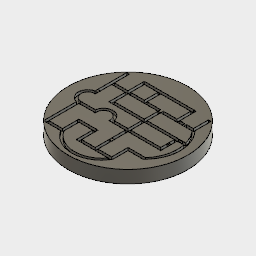
Maze_completed (Autodesk Fusion 360 design; units mm, degrees)
Autodesk Fusion 360 part; units mm, degrees
note: some values were not read from the file. Set by a fixed rule: which sketch regions a step uses.
(part 1 of 2)
sketch "Sketch1" plane through (0, 0, 0) normal (0, 1, 0) x (1, 0, 0)
  circle A0 centre (0, 0) radius 152.4
extrude "Extrude1" add sketch "Sketch1" along normal blind 25.4 makes body 1
sketch "Sketch2" plane through (0, 25.4, 0) normal (0, 1, 0) x (-1, 0, 0)
  circle A0 centre (0, 0) radius 152.4
  line L0 (62.5721, -104.2868) -> (62.572, -20.8574)
  line L1 (62.572, -20.8574) -> (-20.8574, -20.8574)
  line L2 (-20.8574, -20.8574) -> (-20.8574, 20.8573)
  line L3 (-20.8574, 20.8573) -> (20.8573, 20.8573)
  line L4 (62.572, 20.8573) -> (104.2868, 20.8573)
  line L5 (104.2868, 20.8573) -> (104.2868, 62.572)
  line L6 (104.2868, 62.572) -> (104.2868, 104.287)
  line L7 (104.2868, 104.287) -> (62.5718, 104.2869)
  line L8 (-62.5723, 104.2867) -> (-62.5722, 62.572)
  line L9 (-62.5722, 62.572) -> (-104.2867, 62.572)
  arc A1 (-104.2867, 62.572) -> (-104.2867, -62.5721) centre (-41.0104, -0.0001) ccw
  arc A2 (20.8573, 20.8573) -> (62.572, 20.8573) centre (41.7146, 20.7869) ccw
  line L10 (104.2868, -104.2868) -> (104.2868, -20.8574)
  line L11 (20.8572, 62.572) -> (20.8571, 104.2868)
  line L12 (62.5719, 62.572) -> (20.8572, 62.572)
  line L13 (62.5718, 104.2869) -> (62.5719, 62.572)
  line L14 (20.8571, 104.2868) -> (-62.5723, 104.2867)
  line L15 (62.5721, -62.5721) -> (20.8574, -62.5721)
  line L16 (20.8574, -62.5721) -> (20.8574, -104.2868)
  line L17 (20.8574, -104.2868) -> (-20.8573, -104.2868)
  line L18 (-20.8573, -104.2868) -> (-62.572, -104.2868)
  line L19 (-104.2867, -62.5721) -> (-104.2867, -104.2868)
  line L20 (-104.2867, -62.5721) -> (-62.5721, -62.5721)
  line L21 (-62.5721, -62.5721) -> (-20.8573, -62.5721)
  line L22 (-20.8573, -62.5721) -> (-20.8574, -20.8574)
  line L23 (-20.8574, -20.8574) -> (-104.2867, -20.8574)
  line L24 (-104.2867, -20.8574) -> (-127.5212, -20.8575)
  line L25 (-20.8575, 62.572) -> (-20.8574, 20.8573)
  line L26 (-20.8575, 62.572) -> (-20.8576, 104.2868)
  line L27 (-62.5721, 20.8573) -> (-20.8574, 20.8573)
  line L28 (-104.2867, 20.8573) -> (-62.5721, 20.8573)
  line L29 (-104.2867, -20.8574) -> (-104.2867, 20.8573)
  arc A3 (104.2868, -20.8574) -> (104.2868, 20.8573) centre (102.4601, -0.0001) ccw
  line L30 (104.2868, -62.5721) -> (62.5721, -62.5721)
  arc A4 (62.5718, 104.2869) -> (-62.5723, 104.2867) centre (-0.0002, 67.3281) ccw
  circle A5 centre (123.3973, -0.0001) radius 7.4836
  circle A6 centre (-0.0003, 140) radius 10
  circle A7 centre (-104.2867, -0.0001) radius 7.4484
  line L31 (62.5721, -104.2868) -> (20.8574, -104.2868)
  line L32 (-62.572, -104.2868) -> (-62.5721, -62.5721)
  circle A8 centre (-20.8575, 83.4294) radius 6.8677
  circle A9 centre (-83.4294, -62.5721) radius 5.1809
  circle A10 centre (-115.9039, -20.8575) radius 5.6269
  line L33 (20.8574, -62.5721) -> (-20.8573, -62.5721)
  circle A11 centre (-20.8573, -62.5721) radius 8.2188
  line L34 (104.2868, -104.2868) -> (100.9118, -104.2868)
  line L35 (104.2868, -104.2868) -> (107.6618, -104.2868)
  line L36 (100.9118, -104.2868) -> (100.9118, -62.5721)
  line L37 (107.6618, -104.2868) -> (107.6618, -20.2808)
  line L38 (104.2868, -62.5721) -> (104.2868, -65.9471)
  line L39 (104.2868, -62.5721) -> (104.2868, -59.1971)
  line L40 (104.2868, -65.9471) -> (62.5721, -65.9472)
  line L41 (104.2868, -59.1971) -> (62.5721, -59.1972)
  line L42 (100.9118, -62.5721) -> (100.9118, -20.7212)
  line L43 (62.5721, -62.5721) -> (65.9471, -62.5721)
  line L44 (62.5721, -62.5721) -> (59.1971, -62.5721)
  line L45 (59.1971, -62.5721) -> (59.1971, -104.2868)
  line L46 (65.9471, -62.5721) -> (65.9472, -104.2868)
  line L47 (65.9472, -104.2868) -> (62.5721, -104.2868)
  line L48 (59.1971, -62.5721) -> (59.1971, -20.8574)
  line L49 (65.9471, -62.5721) -> (65.9472, -83.4295)
  line L50 (62.572, -20.8574) -> (65.947, -20.8574)
  line L51 (65.9471, -62.5721) -> (65.947, -20.8574)
  line L52 (104.2868, -20.8574) -> (100.9118, -20.8574)
  line L53 (104.2868, -20.8574) -> (104.2868, -24.2324)
  line L54 (104.2868, -20.8574) -> (104.2868, -17.4824)
  line L55 (104.2868, 20.8573) -> (104.2868, 17.4823)
  line L56 (104.2868, 20.8573) -> (104.2868, 24.2323)
  line L57 (123.3973, -0.0001) -> (126.7723, -0.0001)
  arc A12 (104.2868, -24.2324) -> (104.2868, 24.2323) centre (102.4721, -0.0001) ccw
  line L58 (123.3973, -0.0001) -> (120.0223, -0.0001)
  arc A13 (104.2868, -17.4824) -> (104.2868, 17.4823) centre (102.443, -0.0001) ccw
  line L59 (65.9472, -104.2868) -> (65.9472, -100.9118)
  line L60 (65.9472, -104.2868) -> (65.9471, -107.6618)
  line L61 (-62.572, -104.2868) -> (-62.572, -107.6618)
  line L62 (-62.572, -104.2868) -> (-62.572, -100.9118)
  line L63 (65.9471, -107.6618) -> (-62.572, -107.6618)
  line L64 (-62.572, -100.9118) -> (65.9472, -100.9118)
  line L65 (20.8574, -104.2868) -> (24.2324, -104.2868)
  line L66 (20.8574, -104.2868) -> (17.4824, -104.2868)
  line L67 (17.4824, -104.2868) -> (17.4824, -62.5721)
  line L68 (24.2324, -104.2868) -> (24.2324, -62.5721)
  line L69 (62.5721, -65.9472) -> (20.8574, -65.9473)
  line L70 (20.8574, -62.5721) -> (20.8574, -59.1972)
  line L71 (20.8574, -59.1972) -> (62.5721, -59.1972)
  line L72 (20.8574, -59.1972) -> (-20.8573, -59.1973)
  line L73 (-20.8573, -62.5721) -> (-20.8574, -65.9474)
  line L74 (-20.8574, -65.9474) -> (20.8574, -65.9473)
  line L75 (-20.8574, -65.9474) -> (-104.2867, -65.9474)
  line L76 (-20.8573, -59.1973) -> (-104.2867, -59.1973)
  line L77 (-104.2867, -59.1973) -> (-104.2867, -62.5721)
  line L78 (-104.2867, -62.5721) -> (-107.6617, -62.5721)
  line L79 (-107.6617, -62.5721) -> (-107.6617, -104.2871)
  line L80 (-107.6617, -104.2871) -> (-104.2867, -104.2868)
  line L81 (-104.2867, -62.5721) -> (-100.9117, -62.5721)
  line L82 (-100.9117, -62.5721) -> (-100.9117, -104.287)
  line L83 (-100.9117, -104.287) -> (-104.2867, -104.2868)
  line L84 (-104.2867, -59.1973) -> (-107.6617, -59.1973)
  line L85 (-107.6617, -59.1973) -> (-107.6617, -62.5721)
  line L86 (-104.2867, 62.572) -> (-104.2867, 65.947)
  line L87 (-104.2867, -62.5721) -> (-104.2867, -66.5721)
  line L88 (-104.2867, -62.5721) -> (-104.2867, -58.5721)
  line L89 (-104.2867, 62.572) -> (-104.2867, 66.572)
  line L90 (-104.2867, 62.572) -> (-104.2867, 58.572)
  arc A14 (-100.9117, 62.572) -> (-100.9117, -62.5721) centre (-37.6354, -0.0001) ccw
  arc A15 (-107.6617, 62.572) -> (-107.6617, -62.5721) centre (-44.3854, -0.0001) ccw
  line L91 (65.947, -20.8574) -> (65.947, -24.2324)
  line L92 (65.947, -20.8574) -> (65.947, -17.4824)
  line L93 (65.947, -17.4824) -> (-104.2867, -17.4824)
  line L94 (65.947, -24.2324) -> (-104.2867, -24.2329)
  line L95 (-104.2867, -24.2329) -> (-104.2867, -20.8574)
  line L96 (-20.8574, -20.8574) -> (-17.4824, -20.8574)
  line L97 (-20.8574, -20.8574) -> (-24.2324, -20.8574)
  line L98 (-24.2324, -20.8574) -> (-24.2324, -62.5721)
  line L99 (-17.4824, -20.8574) -> (-17.4824, -62.5721)
  line L100 (-104.2867, -24.2329) -> (-123.262, -24.2329)
  line L101 (-104.2867, -17.4824) -> (-124.8909, -17.4824)
  line L102 (20.8573, 20.8573) -> (20.8573, 17.4823)
  line L103 (20.8573, 17.4823) -> (20.8573, 20.8573)
  line L104 (20.8573, 20.8573) -> (20.8573, 24.2323)
  line L105 (-104.2867, 20.8573) -> (-104.2867, 24.2323)
  line L106 (-104.2867, 24.2323) -> (20.8573, 24.2323)
  line L107 (20.8573, 17.4823) -> (-104.2867, 17.4823)
  line L108 (-104.2867, 24.2323) -> (-107.6617, 24.2323)
  line L109 (-107.6617, 24.2323) -> (-104.2867, 24.2323)
  line L110 (-104.2867, 24.2323) -> (-100.9117, 24.2323)
  line L111 (-100.9117, 24.2323) -> (-100.9117, -20.8574)
  line L112 (-107.6617, 24.2323) -> (-107.6616, -20.8574)
  line L113 (62.572, 20.8573) -> (62.572, 17.4823)
  line L114 (62.572, 17.4823) -> (62.572, 20.8573)
  line L115 (62.572, 20.8573) -> (62.5606, 24.2322)
  line L116 (62.5606, 24.2322) -> (104.2868, 24.2323)
  line L117 (104.2868, 17.4823) -> (62.572, 17.4823)
  line L118 (62.572, 20.8573) -> (65.947, 20.8573)
  line L119 (62.572, 20.8573) -> (59.197, 20.8573)
  line L120 (20.8573, 20.8573) -> (17.4823, 20.8573)
  line L121 (20.8573, 20.8573) -> (24.2323, 20.8573)
  line L122 (41.7146, -0.0706) -> (41.7146, 3.3044)
  line L123 (41.7146, 3.3044) -> (41.7146, -0.0706)
  line L124 (41.7146, -0.0706) -> (41.7146, -3.4456)
  arc A16 (17.4823, 20.8573) -> (65.947, 20.8573) centre (41.7146, 20.7869) ccw
  arc A17 (24.2323, 20.8573) -> (59.197, 20.8573) centre (41.7146, 20.7869) ccw
  line L125 (62.5606, 24.2322) -> (59.1856, 24.2322)
  line L126 (59.1856, 24.2322) -> (59.197, 20.8573)
  line L127 (24.2323, 20.8573) -> (24.2323, 24.2322)
  line L128 (24.2323, 24.2322) -> (20.8573, 24.2323)
  line L129 (-17.4824, -20.8574) -> (-17.4824, 20.8573)
  line L130 (-24.2324, -20.8574) -> (-24.2324, 20.8573)
  line L131 (-62.572, -107.6618) -> (-65.947, -107.6618)
  line L132 (-65.947, -107.6618) -> (-62.572, -107.6618)
  line L133 (-62.572, -107.6618) -> (-59.197, -107.6619)
  line L134 (-59.197, -107.6619) -> (-59.197, -65.9474)
  line L135 (-65.947, -107.6618) -> (-65.947, -65.9474)
  line L136 (104.2868, 104.287) -> (107.6618, 104.287)
  line L137 (107.6618, 104.287) -> (104.2868, 104.287)
  line L138 (104.2868, 104.287) -> (100.9118, 104.287)
  line L139 (107.6618, 104.287) -> (107.6618, 20.2806)
  line L140 (100.9118, 104.287) -> (100.9118, 24.2323)
  line L141 (107.6618, 104.287) -> (104.2868, 107.6568)
  line L142 (104.2868, 107.6568) -> (107.6618, 104.287)
  line L143 (62.5718, 104.2869) -> (62.5718, 100.9119)
  line L144 (62.5718, 100.9119) -> (104.2868, 100.9119)
  line L145 (104.2868, 107.6568) -> (60.4548, 107.6568)
  line L146 (62.5718, 104.2869) -> (59.1968, 104.2869)
  line L147 (59.1968, 104.2869) -> (62.5718, 104.2869)
  line L148 (62.5718, 104.2869) -> (65.9468, 104.2869)
  line L149 (-0.0003, 140) -> (-0.0003, 143.375)
  line L150 (-0.0003, 143.375) -> (-0.0003, 141.6875)
  line L151 (-0.0003, 140) -> (-0.0003, 136.625)
  line L152 (-62.5723, 104.2867) -> (-65.9473, 104.2867)
  line L153 (-62.5723, 104.2867) -> (-59.1973, 104.2867)
  arc A18 (65.9468, 104.2869) -> (-65.9473, 104.2867) centre (-0.0002, 68.2001) ccw
  arc A19 (59.1968, 104.2869) -> (-59.1973, 104.2867) centre (-0.0002, 66.274) ccw
  line L154 (62.5719, 62.572) -> (65.9469, 62.572)
  line L155 (65.9469, 62.572) -> (65.9468, 104.2869)
  line L156 (59.1968, 104.2869) -> (59.1969, 62.572)
  line L157 (65.9469, 62.572) -> (65.9469, 59.197)
  line L158 (65.9469, 59.197) -> (65.9469, 62.572)
  line L159 (65.9469, 62.572) -> (65.9469, 65.947)
  line L160 (20.8572, 62.572) -> (20.8571, 59.197)
  line L161 (65.9469, 59.197) -> (20.8571, 59.197)
  line L162 (65.9469, 65.947) -> (20.8572, 65.9469)
  line L163 (20.8571, 59.197) -> (17.4821, 59.197)
  line L164 (17.4821, 59.197) -> (17.4821, 104.2868)
  line L165 (20.8572, 62.572) -> (24.2322, 62.572)
  line L166 (24.2322, 62.572) -> (24.2322, 104.287)
  line L167 (24.2322, 104.287) -> (20.8571, 104.2868)
  line L168 (-17.4824, 20.8573) -> (-17.4825, 104.2868)
  line L169 (-24.2324, 20.8573) -> (-24.2324, 104.2868)
  line L170 (24.2322, 104.287) -> (24.2321, 107.662)
  line L171 (24.2322, 104.287) -> (24.2322, 100.912)
  line L172 (24.2322, 100.912) -> (-62.5723, 100.9118)
  line L173 (24.2321, 107.662) -> (-60.4537, 107.659)
  line L174 (-62.5722, 62.572) -> (-62.5722, 59.197)
  line L175 (-62.5722, 59.197) -> (-104.0798, 59.197)
  line L176 (-104.2867, 65.947) -> (-62.5722, 65.947)
  line L177 (-65.9473, 104.2867) -> (-65.9473, 59.197)
  line L178 (-62.5722, 59.197) -> (-59.1972, 59.197)
  line L179 (-59.1972, 59.197) -> (-59.1973, 104.2867)
  point P0 (62.5721, -104.2868)
  point P1 (62.5721, -62.5721)
  point P2 (62.572, -20.8574)
  point P3 (62.572, 20.8573)
  point P4 (62.5719, 62.572)
  point P5 (62.5718, 104.2869)
  point P6 (20.8571, 104.2868)
  point P7 (20.8572, 62.572)
  point P8 (20.8573, 20.8573)
  point P9 (20.8574, -20.8574)
  point P10 (20.8574, -62.5721)
  point P11 (20.8574, -104.2868)
  point P12 (104.2868, -104.2868)
  point P13 (104.2868, -62.5721)
  point P14 (104.2868, -20.8574)
  point P15 (104.2868, 20.8573)
  point P16 (104.2868, 62.572)
  point P17 (104.2868, 104.287)
  point P18 (-20.8576, 104.2868)
  point P19 (-62.5722, 62.572)
  point P20 (-104.2867, 20.8573)
  point P21 (-62.5721, -20.8574)
  point P22 (-20.8573, -62.5721)
  point P23 (-62.572, -104.2868)
  point P24 (-104.2867, -104.2868)
  point P25 (-20.8573, -104.2868)
  point P26 (-62.5721, -62.5721)
  point P27 (-104.2867, -62.5721)
  point P28 (-104.2867, -20.8574)
  point P29 (-20.8574, -20.8574)
  point P30 (-20.8574, 20.8573)
  point P31 (-62.5721, 20.8573)
  point P32 (-20.8575, 62.572)
  point P33 (-62.5723, 104.2867)
  point P34 (-104.2867, 62.572)
  point P35 (-104.2867, 104.2867)
  dimension "d19" = 3.375
  dimension "d20" = 3.375
  dimension "d21" = 3.375
  dimension "d22" = 3.375
  dimension "d23" = 3.375
  dimension "d24" = 3.375
  dimension "d25" = 3.375
  dimension "d26" = 3.375
  dimension "d27" = 3.375
  dimension "d28" = 3.375
  dimension "d29" = 3.375
  dimension "d30" = 3.375
  dimension "d31" = 3.375
  dimension "d32" = 3.375
  dimension "d33" = 3.375
  dimension "d34" = 3.375
  dimension "d35" = 3.375
  dimension "d36" = 3.375
  dimension "d37" = 3.375
  dimension "d38" = 3.375
  dimension "d39" = 41.715
  dimension "d40" = 3.375
  dimension "d41" = 4
  dimension "d42" = 3.375
  dimension "d43" = 3.375
  dimension "d44" = 3.375
  dimension "d45" = 3.375
  dimension "d46" = 3.375
  dimension "d47" = 3.375
  dimension "d48" = 3.375
  dimension "d49" = 3.375
  dimension "d50" = 3.375
  dimension "d51" = 3.375
  dimension "d52" = 3.375
  dimension "d53" = 3.375
  dimension "d54" = 41.715
  dimension "d55" = 3.375
  dimension "d56" = 3.375
  measures "d19" distance of P12 L34.end
  measures "d20" distance of P12 L35.end
  measures "d21" distance of P13 L38.end
  measures "d22" distance of P13 L39.end
  measures "d23" distance of P1 L43.end
  measures "d24" distance of P1 L44.end
  measures "d25" distance of P2 L50.end
  measures "d26" distance of P14 L52.end
  measures "d27" distance of P14 L53.end
  measures "d28" distance of P14 L54.end
  measures "d29" distance of P15 L55.end
  measures "d30" distance of P15 L56.end
  measures "d31" distance of A5.centre L57.end
  measures "d32" distance of A5.centre L58.end
  measures "d33" distance of L46.end L59.end
  measures "d34" distance of L46.end L60.end
  measures "d35" distance of P23 L61.end
  measures "d36" distance of P23 L62.end
  measures "d37" distance of P11 L65.end
  measures "d38" distance of P11 L66.end
  measures "d39" distance of L78.end L79.end
  measures "d40" distance of P34 L86.end
  measures "d41" distance of P34 L89.end
  measures "d42" distance of P8 L102.end
  measures "d43" distance of P8 L104.end
  measures "d44" distance of L115.end L125.end
  measures "d45" distance of L61.end L133.end
  measures "d46" distance of P17 L138.end
  measures "d47" distance of P5 L143.end
  measures "d48" distance of P5 L148.end
  measures "d49" distance of A6.centre L151.end
  measures "d50" distance of P33 L152.end
  measures "d51" distance of P33 L153.end
  measures "d52" distance of P4 L154.end
  measures "d53" distance of P7 L160.end
  measures "d54" distance of L165.end L166.end
  measures "d55" distance of L166.end L170.end
  measures "d56" distance of P19 L174.end
extrude "Extrude2" add sketch "Sketch2" along normal blind 7 contours A0 | L45 L64 L68 L69 | A5 L41 L42 L51 L52 L54 A13 L91 L92 L93 L107 L117 A16 L129 | A11 L48 L71 L72 L94 L99 | L10 L41 L42 L52 L53 | A11 L64 L67 L74 L75 L134 | A11 L72 L99 | A11 L74 L75 | A9 A10 A11 L76 A14 L94 L98 L100 | A5 A12 | A11 L76 L98 | A5 A13 | A7 L93 L107 L111 L130 | A10 L100 | A9 L75 | A9 L76 | A8 L106 L116 A17 L125 L126 L127 L128 L140 L144 L155 L157 L158 L159 L161 L163 L164 L168 L172 | A7 L111 | A8 L168 | A7 A8 A10 A14 L101 L106 L108 L109 L110 L112 L169 L172 L175 L178 L179 | A10 L101 | A7 L112 | A8 L169 | A6 A18 | A6 A19 L156 L162 L166 L170 L171 L173 | A6 A19 bodies 1
sketch "Sketch3" plane through (0, 32.4, 0) normal (0, 1, 0) x (-1, 0, 0)
  line L0 (63.9876, 107.6568) -> (104.2868, 107.6568)
  line L1 (104.2868, 107.6568) -> (107.6618, 104.287)
  line L2 (107.6618, 104.287) -> (107.6618, 23.7395)
  arc A0 (107.6618, -23.7396) -> (107.6618, 23.7395) centre (102.4721, -0.0001) ccw
  line L3 (107.6618, -23.7396) -> (107.6618, -104.2868)
  line L4 (107.6618, -104.2868) -> (100.9118, -104.2868)
  line L5 (100.9118, -104.2868) -> (100.9118, -65.9471)
  line L6 (100.9118, -65.9471) -> (65.9471, -65.9472)
  line L7 (65.9471, -65.9472) -> (65.9472, -104.2868)
  line L8 (65.9472, -104.2868) -> (65.9471, -107.6618)
  line L9 (65.9471, -107.6618) -> (-59.197, -107.6618)
  line L10 (-59.197, -107.6618) -> (-59.197, -107.6619)
  line L11 (-59.197, -107.6619) -> (-62.572, -107.6618)
  line L12 (-62.572, -107.6618) -> (-65.947, -107.6618)
  line L13 (-65.947, -107.6618) -> (-65.947, -65.9474)
  line L14 (-65.947, -65.9474) -> (-100.9117, -65.9474)
  line L15 (-100.9117, -65.9474) -> (-100.9117, -104.287)
  line L16 (-100.9117, -104.287) -> (-104.2867, -104.2868)
  line L17 (-104.2867, -104.2868) -> (-107.6617, -104.2871)
  line L18 (-107.6617, -104.2871) -> (-107.6617, -59.1973)
  line L19 (-107.6617, -59.1973) -> (-107.4547, -59.1973)
  arc A1 (-104.2867, 62.572) -> (-107.4547, -59.1973) centre (-41.0104, -0.0001) ccw
  line L20 (-104.2867, 62.572) -> (-104.2867, 65.947)
  line L21 (-104.2867, 65.947) -> (-65.9473, 65.947)
  line L22 (-65.9473, 65.947) -> (-65.9473, 104.2867)
  arc A2 (63.9876, 107.6568) -> (-65.9473, 104.2867) centre (-0.0002, 68.2001) ccw
  circle A3 centre (0, 0) radius 152.4
  line L23 (-107.4547, -59.1973) -> (-107.5908, -63.1949)
  arc A4 (-104.2867, 65.947) -> (-107.5908, -63.1949) centre (-42.5552, -0.2457) ccw
  dimension "d59" = 4
  measures "d59" distance of L19.end L23.end
extrude "Extrude3" cut sketch "Sketch3" against normal blind 7 contours L18 L19 A1 L20 A4 bodies 1
sketch "Sketch4" plane through (0, 32.4, 0) normal (0, 1, 0) x (-1, 0, 0)
  line L0 (65.947, -17.4824) -> (65.9471, -59.1972)
  line L1 (65.9471, -59.1972) -> (104.2868, -59.1971)
  line L2 (104.2868, -59.1971) -> (104.2868, -17.4824)
  arc A0 (104.2868, -17.4824) -> (104.2868, 17.4823) centre (102.443, -0.0001) ccw
  line L3 (104.2868, 17.4823) -> (65.7207, 17.4823)
  arc A1 (17.7085, 17.4823) -> (65.7207, 17.4823) centre (41.7146, 20.7869) ccw
  line L4 (17.7085, 17.4823) -> (-17.4824, 17.4823)
  line L5 (-17.4824, 17.4823) -> (-17.4824, -17.4824)
  line L6 (-17.4824, -17.4824) -> (65.947, -17.4824)
  line L7 (104.2868, -17.4824) -> (100.9118, -17.4824)
  line L8 (100.9118, -17.4824) -> (100.9118, -59.1972)
  dimension "d62" = 3.375
  measures "d62" distance of L2.end L7.end
extrude "Extrude4" cut sketch "Sketch4" against normal blind 7 contours L1 L2 L7 L8 bodies 1
sketch "Sketch5" plane through (0, 25.4, 0) normal (0, 1, 0) x (-1, 0, 0)
  line L0 (-20.8574, -65.9474) -> (17.4824, -65.9473)
  line L1 (17.4824, -65.9473) -> (17.4824, -100.9118)
  line L2 (17.4824, -100.9118) -> (-59.197, -100.9118)
  line L3 (-59.197, -100.9118) -> (-59.197, -65.9474)
  line L4 (-59.197, -65.9474) -> (-20.8574, -65.9474)
  line L5 (-59.1972, 59.197) -> (-59.1973, 100.9118)
  line L6 (-59.1973, 100.9118) -> (-24.2324, 100.9119)
  line L7 (-24.2324, 100.9119) -> (-24.2324, 24.2323)
  line L8 (-24.2324, 24.2323) -> (-107.6617, 24.2323)
  line L9 (-107.6617, 24.2323) -> (-107.6616, -17.4824)
  line L10 (-107.6616, -17.4824) -> (-124.8909, -17.4824)
  arc A0 (-104.0798, 59.197) -> (-124.8909, -17.4824) centre (-37.6354, -0.0001) ccw
  line L11 (-104.0798, 59.197) -> (-59.1972, 59.197)
  arc A1 (63.9876, 107.6568) -> (-65.9473, 104.2867) centre (-0.0002, 68.2001) ccw
  line L12 (-65.9473, 104.2867) -> (-65.9473, 65.947)
  line L13 (-65.9473, 65.947) -> (-104.2867, 65.947)
  arc A2 (-104.2867, 65.947) -> (-107.6617, -63.1217) centre (-42.5552, -0.2457) ccw
  line L14 (-107.6617, -63.1217) -> (-107.6617, -104.2871)
  line L15 (-107.6617, -104.2871) -> (-104.2867, -104.2868)
  line L16 (-104.2867, -104.2868) -> (-100.9117, -104.287)
  line L17 (-100.9117, -104.287) -> (-100.9117, -65.9474)
  line L18 (-100.9117, -65.9474) -> (-65.947, -65.9474)
  line L19 (-65.947, -65.9474) -> (-65.947, -107.6618)
  line L20 (-65.947, -107.6618) -> (-62.572, -107.6618)
  line L21 (-62.572, -107.6618) -> (-59.197, -107.6619)
  line L22 (-59.197, -107.6619) -> (-59.197, -107.6618)
  line L23 (-59.197, -107.6618) -> (65.9471, -107.6618)
  line L24 (65.9471, -107.6618) -> (65.9472, -104.2868)
  line L25 (65.9472, -104.2868) -> (65.9471, -65.9472)
  line L26 (65.9471, -65.9472) -> (100.9118, -65.9471)
  line L27 (100.9118, -65.9471) -> (100.9118, -104.2868)
  line L28 (100.9118, -104.2868) -> (107.6618, -104.2868)
  line L29 (107.6618, -104.2868) -> (107.6618, -23.7396)
  arc A3 (107.6618, -23.7396) -> (107.6618, 23.7395) centre (102.4721, -0.0001) ccw
  line L30 (107.6618, 23.7395) -> (107.6618, 104.287)
  line L31 (107.6618, 104.287) -> (104.2868, 107.6568)
  line L32 (104.2868, 107.6568) -> (63.9876, 107.6568)
  line L33 (65.947, -17.4824) -> (-17.4824, -17.4824)
  line L34 (-17.4824, -17.4824) -> (-17.4824, 17.4823)
  line L35 (-17.4824, 17.4823) -> (17.7085, 17.4823)
  arc A4 (17.7085, 17.4823) -> (65.7207, 17.4823) centre (41.7146, 20.7869) ccw
  line L36 (65.7207, 17.4823) -> (104.2868, 17.4823)
  arc A5 (104.2868, -17.4824) -> (104.2868, 17.4823) centre (102.443, -0.0001) ccw
  line L37 (104.2868, -17.4824) -> (100.9118, -17.4824)
  line L38 (100.9118, -17.4824) -> (100.9118, -59.1971)
  line L39 (100.9118, -59.1971) -> (65.9471, -59.1972)
  line L40 (65.9471, -59.1972) -> (65.947, -17.4824)
  line L41 (65.9469, 59.197) -> (65.9469, 62.572)
  line L42 (65.9469, 62.572) -> (65.9468, 100.9119)
  line L43 (65.9468, 100.9119) -> (100.9118, 100.9119)
  line L44 (100.9118, 100.9119) -> (100.9118, 24.2323)
  line L45 (100.9118, 24.2323) -> (62.5606, 24.2322)
  line L46 (62.5606, 24.2322) -> (59.1856, 24.2322)
  line L47 (59.1856, 24.2322) -> (59.197, 20.8573)
  arc A6 (24.2323, 20.8573) -> (59.197, 20.8573) centre (41.7146, 20.7869) ccw
  line L48 (24.2323, 20.8573) -> (24.2323, 24.2322)
  line L49 (24.2323, 24.2322) -> (20.8573, 24.2323)
  line L50 (20.8573, 24.2323) -> (-17.4824, 24.2323)
  line L51 (-17.4824, 24.2323) -> (-17.4825, 100.9119)
  line L52 (-17.4825, 100.9119) -> (17.4821, 100.912)
  line L53 (17.4821, 100.912) -> (17.4821, 59.197)
  line L54 (17.4821, 59.197) -> (20.8571, 59.197)
  line L55 (20.8571, 59.197) -> (65.9469, 59.197)
  line L56 (20.8574, -59.1972) -> (-17.4824, -59.1973)
  line L57 (-17.4824, -59.1973) -> (-17.4824, -24.2327)
  line L58 (-17.4824, -24.2327) -> (59.1971, -24.2325)
  line L59 (59.1971, -24.2325) -> (59.1971, -59.1972)
  line L60 (59.1971, -59.1972) -> (20.8574, -59.1972)
  line L61 (-24.2324, 17.4823) -> (-24.2324, -17.4824)
  line L62 (-24.2324, -17.4824) -> (-100.9117, -17.4824)
  line L63 (-100.9117, -17.4824) -> (-100.9117, 17.4823)
  line L64 (-100.9117, 17.4823) -> (-24.2324, 17.4823)
  line L65 (24.2324, -100.9118) -> (24.2324, -65.9473)
  line L66 (24.2324, -65.9473) -> (59.1971, -65.9472)
  line L67 (59.1971, -65.9472) -> (59.1971, -100.9118)
  line L68 (59.1971, -100.9118) -> (24.2324, -100.9118)
  line L69 (24.2322, 104.287) -> (24.2321, 107.662)
  line L70 (24.2321, 107.662) -> (-56.8908, 107.6591)
  arc A7 (59.1968, 104.2869) -> (-56.8908, 107.6591) centre (-0.0002, 66.274) ccw
  line L71 (59.1968, 104.2869) -> (59.1969, 65.947)
  line L72 (59.1969, 65.947) -> (24.2322, 65.9469)
  line L73 (24.2322, 65.9469) -> (24.2322, 104.287)
  line L74 (-24.2324, -24.2327) -> (-24.2324, -59.1973)
  line L75 (-24.2324, -59.1973) -> (-104.0797, -59.1973)
  arc A8 (-123.262, -24.2329) -> (-104.0797, -59.1973) centre (-37.6354, -0.0001) ccw
  line L76 (-123.262, -24.2329) -> (-104.2867, -24.2329)
  line L77 (-104.2867, -24.2329) -> (-24.2324, -24.2327)
  line L78 (100.9118, 24.2323) -> (96.9118, 24.2323)
  line L79 (96.9118, 24.2323) -> (96.9118, 17.4823)
  line L80 (96.9118, 17.4823) -> (100.9118, 17.4823)
  line L81 (100.9118, 17.4823) -> (100.9118, 24.2323)
extrude "Extrude5" add sketch "Sketch5" along normal blind 7 contours L36 L45 L78 L79 L80 L81 bodies 1
sketch "Sketch6" plane through (0, 25.4, 0) normal (0, 1, 0) x (-1, 0, 0)
  line L0 (-24.2324, -24.2327) -> (-24.2324, -59.1973)
  line L1 (-24.2324, -59.1973) -> (-104.0797, -59.1973)
  arc A0 (-123.262, -24.2329) -> (-104.0797, -59.1973) centre (-37.6354, -0.0001) ccw
  line L2 (-123.262, -24.2329) -> (-104.2867, -24.2329)
  line L3 (-104.2867, -24.2329) -> (-24.2324, -24.2327)
  line L4 (24.2322, 104.287) -> (24.2321, 107.662)
  line L5 (24.2321, 107.662) -> (-56.8908, 107.6591)
  arc A1 (59.1968, 104.2869) -> (-56.8908, 107.6591) centre (-0.0002, 66.274) ccw
  line L6 (59.1968, 104.2869) -> (59.1969, 65.947)
  line L7 (59.1969, 65.947) -> (24.2322, 65.9469)
  line L8 (24.2322, 65.9469) -> (24.2322, 104.287)
  line L9 (24.2324, -100.9118) -> (24.2324, -65.9473)
  line L10 (24.2324, -65.9473) -> (59.1971, -65.9472)
  line L11 (59.1971, -65.9472) -> (59.1971, -100.9118)
  line L12 (59.1971, -100.9118) -> (24.2324, -100.9118)
  line L13 (-24.2324, 17.4823) -> (-24.2324, -17.4824)
  line L14 (-24.2324, -17.4824) -> (-100.9117, -17.4824)
  line L15 (-100.9117, -17.4824) -> (-100.9117, 17.4823)
  line L16 (-100.9117, 17.4823) -> (-24.2324, 17.4823)
  line L17 (20.8574, -59.1972) -> (-17.4824, -59.1973)
  line L18 (-17.4824, -59.1973) -> (-17.4824, -24.2327)
  line L19 (-17.4824, -24.2327) -> (59.1971, -24.2325)
  line L20 (59.1971, -24.2325) -> (59.1971, -59.1972)
  line L21 (59.1971, -59.1972) -> (20.8574, -59.1972)
  line L22 (96.9118, 17.4823) -> (96.9118, 24.2323)
  line L23 (96.9118, 24.2323) -> (62.5606, 24.2322)
  line L24 (62.5606, 24.2322) -> (59.1856, 24.2322)
  line L25 (59.1856, 24.2322) -> (59.197, 20.8573)
  arc A2 (24.2323, 20.8573) -> (59.197, 20.8573) centre (41.7146, 20.7869) ccw
  line L26 (24.2323, 20.8573) -> (24.2323, 24.2322)
  line L27 (24.2323, 24.2322) -> (20.8573, 24.2323)
  line L28 (20.8573, 24.2323) -> (-17.4824, 24.2323)
  line L29 (-17.4824, 24.2323) -> (-17.4825, 100.9119)
  line L30 (-17.4825, 100.9119) -> (17.4821, 100.912)
  line L31 (17.4821, 100.912) -> (17.4821, 59.197)
  line L32 (17.4821, 59.197) -> (20.8571, 59.197)
  line L33 (20.8571, 59.197) -> (65.9469, 59.197)
  line L34 (65.9469, 59.197) -> (65.9469, 62.572)
  line L35 (65.9469, 62.572) -> (65.9468, 100.9119)
  line L36 (65.9468, 100.9119) -> (100.9118, 100.9119)
  line L37 (100.9118, 100.9119) -> (100.9118, 17.4823)
  line L38 (100.9118, 17.4823) -> (104.2868, 17.4823)
  arc A3 (104.2868, -17.4824) -> (104.2868, 17.4823) centre (102.443, -0.0001) ccw
  line L39 (104.2868, -17.4824) -> (100.9118, -17.4824)
  line L40 (100.9118, -17.4824) -> (100.9118, -59.1971)
  line L41 (100.9118, -59.1971) -> (65.9471, -59.1972)
  line L42 (65.9471, -59.1972) -> (65.947, -17.4824)
  line L43 (65.947, -17.4824) -> (-17.4824, -17.4824)
  line L44 (-17.4824, -17.4824) -> (-17.4824, 17.4823)
  line L45 (-17.4824, 17.4823) -> (17.7085, 17.4823)
  arc A4 (17.7085, 17.4823) -> (65.7207, 17.4823) centre (41.7146, 20.7869) ccw
  line L46 (65.7207, 17.4823) -> (96.9118, 17.4823)
  arc A5 (63.9876, 107.6568) -> (-65.9473, 104.2867) centre (-0.0002, 68.2001) ccw
  line L47 (-65.9473, 104.2867) -> (-65.9473, 65.947)
  line L48 (-65.9473, 65.947) -> (-104.2867, 65.947)
  arc A6 (-104.2867, 65.947) -> (-107.6617, -63.1217) centre (-42.5552, -0.2457) ccw
  line L49 (-107.6617, -63.1217) -> (-107.6617, -104.2871)
  line L50 (-107.6617, -104.2871) -> (-104.2867, -104.2868)
  line L51 (-104.2867, -104.2868) -> (-100.9117, -104.287)
  line L52 (-100.9117, -104.287) -> (-100.9117, -65.9474)
  line L53 (-100.9117, -65.9474) -> (-65.947, -65.9474)
  line L54 (-65.947, -65.9474) -> (-65.947, -107.6618)
  line L55 (-65.947, -107.6618) -> (-62.572, -107.6618)
  line L56 (-62.572, -107.6618) -> (-59.197, -107.6619)
  line L57 (-59.197, -107.6619) -> (-59.197, -107.6618)
  line L58 (-59.197, -107.6618) -> (65.9471, -107.6618)
  line L59 (65.9471, -107.6618) -> (65.9472, -104.2868)
  line L60 (65.9472, -104.2868) -> (65.9471, -65.9472)
  line L61 (65.9471, -65.9472) -> (100.9118, -65.9471)
  line L62 (100.9118, -65.9471) -> (100.9118, -104.2868)
  line L63 (100.9118, -104.2868) -> (107.6618, -104.2868)
  line L64 (107.6618, -104.2868) -> (107.6618, -23.7396)
  arc A7 (107.6618, -23.7396) -> (107.6618, 23.7395) centre (102.4721, -0.0001) ccw
  line L65 (107.6618, 23.7395) -> (107.6618, 104.287)
  line L66 (107.6618, 104.287) -> (104.2868, 107.6568)
  line L67 (104.2868, 107.6568) -> (63.9876, 107.6568)
  line L68 (-59.1972, 59.197) -> (-59.1973, 100.9118)
  line L69 (-59.1973, 100.9118) -> (-24.2324, 100.9119)
  line L70 (-24.2324, 100.9119) -> (-24.2324, 24.2323)
  line L71 (-24.2324, 24.2323) -> (-107.6617, 24.2323)
  line L72 (-107.6617, 24.2323) -> (-107.6616, -17.4824)
  line L73 (-107.6616, -17.4824) -> (-124.8909, -17.4824)
  arc A8 (-104.0798, 59.197) -> (-124.8909, -17.4824) centre (-37.6354, -0.0001) ccw
  line L74 (-104.0798, 59.197) -> (-59.1972, 59.197)
  line L75 (-20.8574, -65.9474) -> (17.4824, -65.9473)
  line L76 (17.4824, -65.9473) -> (17.4824, -100.9118)
  line L77 (17.4824, -100.9118) -> (-59.197, -100.9118)
  line L78 (-59.197, -100.9118) -> (-59.197, -65.9474)
  line L79 (-59.197, -65.9474) -> (-20.8574, -65.9474)
  line L80 (107.6618, 23.7395) -> (100.9118, 23.7395)
  line L81 (100.9118, 23.7395) -> (100.9118, 27.7395)
  line L82 (100.9118, 27.7395) -> (107.6618, 27.7395)
  line L83 (107.6618, 27.7395) -> (107.6618, 23.7395)
  dimension "d67" = 4
  measures "d67" distance of A7.end L82.end
extrude "Extrude6" add sketch "Sketch6" along normal blind 7 contours L37 L65 L80 L81 L82 L83 bodies 1
sketch "Sketch7" plane through (0, 25.4, 0) normal (0, 1, 0) x (-1, 0, 0)
  line L0 (107.6618, 23.7395) -> (100.9118, 23.7395)
  line L1 (100.9118, 23.7395) -> (100.9118, 17.4823)
  line L2 (100.9118, 17.4823) -> (104.2868, 17.4823)
  arc A0 (104.2868, -17.4824) -> (104.2868, 17.4823) centre (102.443, -0.0001) ccw
  line L3 (104.2868, -17.4824) -> (100.9118, -17.4824)
  line L4 (100.9118, -17.4824) -> (100.9118, -59.1971)
  line L5 (100.9118, -59.1971) -> (65.9471, -59.1972)
  line L6 (65.9471, -59.1972) -> (65.947, -17.4824)
  line L7 (65.947, -17.4824) -> (-17.4824, -17.4824)
  line L8 (-17.4824, -17.4824) -> (-17.4824, 17.4823)
  line L9 (-17.4824, 17.4823) -> (17.7085, 17.4823)
  arc A1 (17.7085, 17.4823) -> (65.7207, 17.4823) centre (41.7146, 20.7869) ccw
  line L10 (65.7207, 17.4823) -> (96.9118, 17.4823)
  line L11 (96.9118, 17.4823) -> (96.9118, 24.2323)
  line L12 (96.9118, 24.2323) -> (62.5606, 24.2322)
  line L13 (62.5606, 24.2322) -> (59.1856, 24.2322)
  line L14 (59.1856, 24.2322) -> (59.197, 20.8573)
  arc A2 (24.2323, 20.8573) -> (59.197, 20.8573) centre (41.7146, 20.7869) ccw
  line L15 (24.2323, 20.8573) -> (24.2323, 24.2322)
  line L16 (24.2323, 24.2322) -> (20.8573, 24.2323)
  line L17 (20.8573, 24.2323) -> (-17.4824, 24.2323)
  line L18 (-17.4824, 24.2323) -> (-17.4825, 100.9119)
  line L19 (-17.4825, 100.9119) -> (17.4821, 100.912)
  line L20 (17.4821, 100.912) -> (17.4821, 59.197)
  line L21 (17.4821, 59.197) -> (20.8571, 59.197)
  line L22 (20.8571, 59.197) -> (65.9469, 59.197)
  line L23 (65.9469, 59.197) -> (65.9469, 62.572)
  line L24 (65.9469, 62.572) -> (65.9468, 100.9119)
  line L25 (65.9468, 100.9119) -> (100.9118, 100.9119)
  line L26 (100.9118, 100.9119) -> (100.9118, 27.7395)
  line L27 (100.9118, 27.7395) -> (107.6618, 27.7395)
  line L28 (107.6618, 27.7395) -> (107.6618, 104.287)
  line L29 (107.6618, 104.287) -> (104.2868, 107.6568)
  line L30 (104.2868, 107.6568) -> (63.9876, 107.6568)
  arc A3 (63.9876, 107.6568) -> (-65.9473, 104.2867) centre (-0.0002, 68.2001) ccw
  line L31 (-65.9473, 104.2867) -> (-65.9473, 65.947)
  line L32 (-65.9473, 65.947) -> (-104.2867, 65.947)
  arc A4 (-104.2867, 65.947) -> (-107.6617, -63.1217) centre (-42.5552, -0.2457) ccw
  line L33 (-107.6617, -63.1217) -> (-107.6617, -104.2871)
  line L34 (-107.6617, -104.2871) -> (-104.2867, -104.2868)
  line L35 (-104.2867, -104.2868) -> (-100.9117, -104.287)
  line L36 (-100.9117, -104.287) -> (-100.9117, -65.9474)
  line L37 (-100.9117, -65.9474) -> (-65.947, -65.9474)
  line L38 (-65.947, -65.9474) -> (-65.947, -107.6618)
  line L39 (-65.947, -107.6618) -> (-62.572, -107.6618)
  line L40 (-62.572, -107.6618) -> (-59.197, -107.6619)
  line L41 (-59.197, -107.6619) -> (-59.197, -107.6618)
  line L42 (-59.197, -107.6618) -> (65.9471, -107.6618)
  line L43 (65.9471, -107.6618) -> (65.9472, -104.2868)
  line L44 (65.9472, -104.2868) -> (65.9471, -65.9472)
  line L45 (65.9471, -65.9472) -> (100.9118, -65.9471)
  line L46 (100.9118, -65.9471) -> (100.9118, -104.2868)
  line L47 (100.9118, -104.2868) -> (107.6618, -104.2868)
  line L48 (107.6618, -104.2868) -> (107.6618, -23.7396)
  arc A5 (107.6618, -23.7396) -> (107.6618, 23.7395) centre (102.4721, -0.0001) ccw
  line L49 (-24.2324, -24.2327) -> (-24.2324, -59.1973)
  line L50 (-24.2324, -59.1973) -> (-104.0797, -59.1973)
  arc A6 (-123.262, -24.2329) -> (-104.0797, -59.1973) centre (-37.6354, -0.0001) ccw
  line L51 (-123.262, -24.2329) -> (-104.2867, -24.2329)
  line L52 (-104.2867, -24.2329) -> (-24.2324, -24.2327)
  line L53 (24.2322, 104.287) -> (24.2321, 107.662)
  line L54 (24.2321, 107.662) -> (-56.8908, 107.6591)
  arc A7 (59.1968, 104.2869) -> (-56.8908, 107.6591) centre (-0.0002, 66.274) ccw
  line L55 (59.1968, 104.2869) -> (59.1969, 65.947)
  line L56 (59.1969, 65.947) -> (24.2322, 65.9469)
  line L57 (24.2322, 65.9469) -> (24.2322, 104.287)
  line L58 (24.2324, -100.9118) -> (24.2324, -65.9473)
  line L59 (24.2324, -65.9473) -> (59.1971, -65.9472)
  line L60 (59.1971, -65.9472) -> (59.1971, -100.9118)
  line L61 (59.1971, -100.9118) -> (24.2324, -100.9118)
  line L62 (-24.2324, 17.4823) -> (-24.2324, -17.4824)
  line L63 (-24.2324, -17.4824) -> (-100.9117, -17.4824)
  line L64 (-100.9117, -17.4824) -> (-100.9117, 17.4823)
  line L65 (-100.9117, 17.4823) -> (-24.2324, 17.4823)
  line L66 (20.8574, -59.1972) -> (-17.4824, -59.1973)
  line L67 (-17.4824, -59.1973) -> (-17.4824, -24.2327)
  line L68 (-17.4824, -24.2327) -> (59.1971, -24.2325)
  line L69 (59.1971, -24.2325) -> (59.1971, -59.1972)
  line L70 (59.1971, -59.1972) -> (20.8574, -59.1972)
  line L71 (-59.1972, 59.197) -> (-59.1973, 100.9118)
  line L72 (-59.1973, 100.9118) -> (-24.2324, 100.9119)
  line L73 (-24.2324, 100.9119) -> (-24.2324, 24.2323)
  line L74 (-24.2324, 24.2323) -> (-107.6617, 24.2323)
  line L75 (-107.6617, 24.2323) -> (-107.6616, -17.4824)
  line L76 (-107.6616, -17.4824) -> (-124.8909, -17.4824)
  arc A8 (-104.0798, 59.197) -> (-124.8909, -17.4824) centre (-37.6354, -0.0001) ccw
  line L77 (-104.0798, 59.197) -> (-59.1972, 59.197)
  line L78 (-20.8574, -65.9474) -> (17.4824, -65.9473)
  line L79 (17.4824, -65.9473) -> (17.4824, -100.9118)
  line L80 (17.4824, -100.9118) -> (-59.197, -100.9118)
  line L81 (-59.197, -100.9118) -> (-59.197, -65.9474)
  line L82 (-59.197, -65.9474) -> (-20.8574, -65.9474)
  line L83 (-17.4824, -59.1973) -> (-24.3061, -59.1973)
  line L84 (-24.3061, -59.1973) -> (-24.3061, -65.9474)
  line L85 (-24.3061, -65.9474) -> (-17.4824, -65.9474)
  line L86 (-17.4824, -65.9474) -> (-17.4824, -59.1973)
extrude "Extrude7" cut sketch "Sketch7" along normal blind 7 contours L50 L78 L82 L83 L84 L85 L86 bodies 1
sketch "Sketch8" plane through (0, 25.4, 0) normal (0, 1, 0) x (-1, 0, 0)
  line L0 (-17.4824, -59.1973) -> (-17.4824, -24.2327)
  line L1 (-17.4824, -24.2327) -> (59.1971, -24.2325)
  line L2 (59.1971, -24.2325) -> (59.1971, -59.1972)
  line L3 (59.1971, -59.1972) -> (20.8574, -59.1972)
  line L4 (20.8574, -59.1972) -> (-17.4824, -59.1973)
  line L5 (-17.4824, -65.9474) -> (17.4824, -65.9473)
  line L6 (17.4824, -65.9473) -> (17.4824, -100.9118)
  line L7 (17.4824, -100.9118) -> (-59.197, -100.9118)
  line L8 (-59.197, -100.9118) -> (-59.197, -65.9474)
  line L9 (-59.197, -65.9474) -> (-17.4824, -65.9474)
  line L10 (-17.4824, -65.9474) -> (-17.4824, -65.9474)
  line L11 (-24.2324, -59.1973) -> (-24.3061, -59.1973)
  line L12 (-24.3061, -59.1973) -> (-104.0797, -59.1973)
  arc A0 (-123.262, -24.2329) -> (-104.0797, -59.1973) centre (-37.6354, -0.0001) ccw
  line L13 (-123.262, -24.2329) -> (-104.2867, -24.2329)
  line L14 (-104.2867, -24.2329) -> (-24.2324, -24.2327)
  line L15 (-24.2324, -24.2327) -> (-24.2324, -59.1973)
  line L16 (107.6618, 23.7395) -> (100.9118, 23.7395)
  line L17 (100.9118, 23.7395) -> (100.9118, 17.4823)
  line L18 (100.9118, 17.4823) -> (104.2868, 17.4823)
  arc A1 (104.2868, -17.4824) -> (104.2868, 17.4823) centre (102.443, -0.0001) ccw
  line L19 (104.2868, -17.4824) -> (100.9118, -17.4824)
  line L20 (100.9118, -17.4824) -> (100.9118, -59.1971)
  line L21 (100.9118, -59.1971) -> (65.9471, -59.1972)
  line L22 (65.9471, -59.1972) -> (65.947, -17.4824)
  line L23 (65.947, -17.4824) -> (-17.4824, -17.4824)
  line L24 (-17.4824, -17.4824) -> (-17.4824, 17.4823)
  line L25 (-17.4824, 17.4823) -> (17.7085, 17.4823)
  arc A2 (17.7085, 17.4823) -> (65.7207, 17.4823) centre (41.7146, 20.7869) ccw
  line L26 (65.7207, 17.4823) -> (96.9118, 17.4823)
  line L27 (96.9118, 17.4823) -> (96.9118, 24.2323)
  line L28 (96.9118, 24.2323) -> (62.5606, 24.2322)
  line L29 (62.5606, 24.2322) -> (59.1856, 24.2322)
  line L30 (59.1856, 24.2322) -> (59.197, 20.8573)
  arc A3 (24.2323, 20.8573) -> (59.197, 20.8573) centre (41.7146, 20.7869) ccw
  line L31 (24.2323, 20.8573) -> (24.2323, 24.2322)
  line L32 (24.2323, 24.2322) -> (20.8573, 24.2323)
  line L33 (20.8573, 24.2323) -> (-17.4824, 24.2323)
  line L34 (-17.4824, 24.2323) -> (-17.4825, 100.9119)
  line L35 (-17.4825, 100.9119) -> (17.4821, 100.912)
  line L36 (17.4821, 100.912) -> (17.4821, 59.197)
  line L37 (17.4821, 59.197) -> (20.8571, 59.197)
  line L38 (20.8571, 59.197) -> (65.9469, 59.197)
  line L39 (65.9469, 59.197) -> (65.9469, 62.572)
  line L40 (65.9469, 62.572) -> (65.9468, 100.9119)
  line L41 (65.9468, 100.9119) -> (100.9118, 100.9119)
  line L42 (100.9118, 100.9119) -> (100.9118, 27.7395)
  line L43 (100.9118, 27.7395) -> (107.6618, 27.7395)
  line L44 (107.6618, 27.7395) -> (107.6618, 104.287)
  line L45 (107.6618, 104.287) -> (104.2868, 107.6568)
  line L46 (104.2868, 107.6568) -> (63.9876, 107.6568)
  arc A4 (63.9876, 107.6568) -> (-65.9473, 104.2867) centre (-0.0002, 68.2001) ccw
  line L47 (-65.9473, 104.2867) -> (-65.9473, 65.947)
  line L48 (-65.9473, 65.947) -> (-104.2867, 65.947)
  arc A5 (-104.2867, 65.947) -> (-107.6617, -63.1217) centre (-42.5552, -0.2457) ccw
  line L49 (-107.6617, -63.1217) -> (-107.6617, -104.2871)
  line L50 (-107.6617, -104.2871) -> (-104.2867, -104.2868)
  line L51 (-104.2867, -104.2868) -> (-100.9117, -104.287)
  line L52 (-100.9117, -104.287) -> (-100.9117, -65.9474)
  line L53 (-100.9117, -65.9474) -> (-65.947, -65.9474)
  line L54 (-65.947, -65.9474) -> (-65.947, -107.6618)
  line L55 (-65.947, -107.6618) -> (-62.572, -107.6618)
  line L56 (-62.572, -107.6618) -> (-59.197, -107.6619)
  line L57 (-59.197, -107.6619) -> (-59.197, -107.6618)
  line L58 (-59.197, -107.6618) -> (65.9471, -107.6618)
  line L59 (65.9471, -107.6618) -> (65.9472, -104.2868)
  line L60 (65.9472, -104.2868) -> (65.9471, -65.9472)
  line L61 (65.9471, -65.9472) -> (100.9118, -65.9471)
  line L62 (100.9118, -65.9471) -> (100.9118, -104.2868)
  line L63 (100.9118, -104.2868) -> (107.6618, -104.2868)
  line L64 (107.6618, -104.2868) -> (107.6618, -23.7396)
  arc A6 (107.6618, -23.7396) -> (107.6618, 23.7395) centre (102.4721, -0.0001) ccw
  line L65 (24.2322, 104.287) -> (24.2321, 107.662)
  line L66 (24.2321, 107.662) -> (-56.8908, 107.6591)
  arc A7 (59.1968, 104.2869) -> (-56.8908, 107.6591) centre (-0.0002, 66.274) ccw
  line L67 (59.1968, 104.2869) -> (59.1969, 65.947)
  line L68 (59.1969, 65.947) -> (24.2322, 65.9469)
  line L69 (24.2322, 65.9469) -> (24.2322, 104.287)
  line L70 (24.2324, -100.9118) -> (24.2324, -65.9473)
  line L71 (24.2324, -65.9473) -> (59.1971, -65.9472)
  line L72 (59.1971, -65.9472) -> (59.1971, -100.9118)
  line L73 (59.1971, -100.9118) -> (24.2324, -100.9118)
  line L74 (-24.2324, 17.4823) -> (-24.2324, -17.4824)
  line L75 (-24.2324, -17.4824) -> (-100.9117, -17.4824)
  line L76 (-100.9117, -17.4824) -> (-100.9117, 17.4823)
  line L77 (-100.9117, 17.4823) -> (-24.2324, 17.4823)
  line L78 (-59.1972, 59.197) -> (-59.1973, 100.9118)
  line L79 (-59.1973, 100.9118) -> (-24.2324, 100.9119)
  line L80 (-24.2324, 100.9119) -> (-24.2324, 24.2323)
  line L81 (-24.2324, 24.2323) -> (-107.6617, 24.2323)
  line L82 (-107.6617, 24.2323) -> (-107.6616, -17.4824)
  line L83 (-107.6616, -17.4824) -> (-124.8909, -17.4824)
  arc A8 (-104.0798, 59.197) -> (-124.8909, -17.4824) centre (-37.6354, -0.0001) ccw
  line L84 (-104.0798, 59.197) -> (-59.1972, 59.197)
  line L85 (-17.4824, -59.1973) -> (-24.313, -59.1973)
  line L86 (-24.313, -59.1973) -> (-24.313, -65.9474)
  line L87 (-24.313, -65.9474) -> (-17.4824, -65.9474)
  line L88 (-17.4824, -65.9474) -> (-17.4824, -59.1973)
extrude "Extrude8" add sketch "Sketch8" along normal blind 7 separate body contours L9 L11 L12 L85 L86 L87 L88 makes body 2
sketch "Sketch9" plane through (0, 25.4, 0) normal (0, 1, 0) x (-1, 0, 0)
  line L0 (-17.4824, -59.1973) -> (-17.4824, -24.2327)
  line L1 (-17.4824, -24.2327) -> (59.1971, -24.2325)
  line L2 (59.1971, -24.2325) -> (59.1971, -59.1972)
  line L3 (59.1971, -59.1972) -> (20.8574, -59.1972)
  line L4 (20.8574, -59.1972) -> (-17.4824, -59.1973)
  line L5 (-17.4824, -65.9474) -> (17.4824, -65.9473)
  line L6 (17.4824, -65.9473) -> (17.4824, -100.9118)
  line L7 (17.4824, -100.9118) -> (-59.197, -100.9118)
  line L8 (-59.197, -100.9118) -> (-59.197, -65.9474)
  line L9 (-59.197, -65.9474) -> (-17.4824, -65.9474)
  line L10 (-17.4824, -65.9474) -> (-17.4824, -65.9474)
  line L11 (-24.2324, -59.1973) -> (-24.3061, -59.1973)
  line L12 (-24.3061, -59.1973) -> (-104.0797, -59.1973)
  arc A0 (-123.262, -24.2329) -> (-104.0797, -59.1973) centre (-37.6354, -0.0001) ccw
  line L13 (-123.262, -24.2329) -> (-104.2867, -24.2329)
  line L14 (-104.2867, -24.2329) -> (-24.2324, -24.2327)
  line L15 (-24.2324, -24.2327) -> (-24.2324, -59.1973)
  line L16 (107.6618, 23.7395) -> (100.9118, 23.7395)
  line L17 (100.9118, 23.7395) -> (100.9118, 17.4823)
  line L18 (100.9118, 17.4823) -> (104.2868, 17.4823)
  arc A1 (104.2868, -17.4824) -> (104.2868, 17.4823) centre (102.443, -0.0001) ccw
  line L19 (104.2868, -17.4824) -> (100.9118, -17.4824)
  line L20 (100.9118, -17.4824) -> (100.9118, -59.1971)
  line L21 (100.9118, -59.1971) -> (65.9471, -59.1972)
  line L22 (65.9471, -59.1972) -> (65.947, -17.4824)
  line L23 (65.947, -17.4824) -> (-17.4824, -17.4824)
  line L24 (-17.4824, -17.4824) -> (-17.4824, 17.4823)
  line L25 (-17.4824, 17.4823) -> (17.7085, 17.4823)
  arc A2 (17.7085, 17.4823) -> (65.7207, 17.4823) centre (41.7146, 20.7869) ccw
  line L26 (65.7207, 17.4823) -> (96.9118, 17.4823)
  line L27 (96.9118, 17.4823) -> (96.9118, 24.2323)
  line L28 (96.9118, 24.2323) -> (62.5606, 24.2322)
  line L29 (62.5606, 24.2322) -> (59.1856, 24.2322)
  line L30 (59.1856, 24.2322) -> (59.197, 20.8573)
  arc A3 (24.2323, 20.8573) -> (59.197, 20.8573) centre (41.7146, 20.7869) ccw
  line L31 (24.2323, 20.8573) -> (24.2323, 24.2322)
  line L32 (24.2323, 24.2322) -> (20.8573, 24.2323)
  line L33 (20.8573, 24.2323) -> (-17.4824, 24.2323)
  line L34 (-17.4824, 24.2323) -> (-17.4825, 100.9119)
  line L35 (-17.4825, 100.9119) -> (17.4821, 100.912)
  line L36 (17.4821, 100.912) -> (17.4821, 59.197)
  line L37 (17.4821, 59.197) -> (20.8571, 59.197)
  line L38 (20.8571, 59.197) -> (65.9469, 59.197)
  line L39 (65.9469, 59.197) -> (65.9469, 62.572)
  line L40 (65.9469, 62.572) -> (65.9468, 100.9119)
  line L41 (65.9468, 100.9119) -> (100.9118, 100.9119)
  line L42 (100.9118, 100.9119) -> (100.9118, 27.7395)
  line L43 (100.9118, 27.7395) -> (107.6618, 27.7395)
  line L44 (107.6618, 27.7395) -> (107.6618, 104.287)
  line L45 (107.6618, 104.287) -> (104.2868, 107.6568)
  line L46 (104.2868, 107.6568) -> (63.9876, 107.6568)
  arc A4 (63.9876, 107.6568) -> (-65.9473, 104.2867) centre (-0.0002, 68.2001) ccw
  line L47 (-65.9473, 104.2867) -> (-65.9473, 65.947)
  line L48 (-65.9473, 65.947) -> (-104.2867, 65.947)
  arc A5 (-104.2867, 65.947) -> (-107.6617, -63.1217) centre (-42.5552, -0.2457) ccw
  line L49 (-107.6617, -63.1217) -> (-107.6617, -104.2871)
  line L50 (-107.6617, -104.2871) -> (-104.2867, -104.2868)
  line L51 (-104.2867, -104.2868) -> (-100.9117, -104.287)
  line L52 (-100.9117, -104.287) -> (-100.9117, -65.9474)
  line L53 (-100.9117, -65.9474) -> (-65.947, -65.9474)
  line L54 (-65.947, -65.9474) -> (-65.947, -107.6618)
  line L55 (-65.947, -107.6618) -> (-62.572, -107.6618)
  line L56 (-62.572, -107.6618) -> (-59.197, -107.6619)
  line L57 (-59.197, -107.6619) -> (-59.197, -107.6618)
  line L58 (-59.197, -107.6618) -> (65.9471, -107.6618)
  line L59 (65.9471, -107.6618) -> (65.9472, -104.2868)
  line L60 (65.9472, -104.2868) -> (65.9471, -65.9472)
  line L61 (65.9471, -65.9472) -> (100.9118, -65.9471)
  line L62 (100.9118, -65.9471) -> (100.9118, -104.2868)
  line L63 (100.9118, -104.2868) -> (107.6618, -104.2868)
  line L64 (107.6618, -104.2868) -> (107.6618, -23.7396)
  arc A6 (107.6618, -23.7396) -> (107.6618, 23.7395) centre (102.4721, -0.0001) ccw
  line L65 (24.2322, 104.287) -> (24.2321, 107.662)
  line L66 (24.2321, 107.662) -> (-56.8908, 107.6591)
  arc A7 (59.1968, 104.2869) -> (-56.8908, 107.6591) centre (-0.0002, 66.274) ccw
  line L67 (59.1968, 104.2869) -> (59.1969, 65.947)
  line L68 (59.1969, 65.947) -> (24.2322, 65.9469)
  line L69 (24.2322, 65.9469) -> (24.2322, 104.287)
  line L70 (24.2324, -100.9118) -> (24.2324, -65.9473)
  line L71 (24.2324, -65.9473) -> (59.1971, -65.9472)
  line L72 (59.1971, -65.9472) -> (59.1971, -100.9118)
  line L73 (59.1971, -100.9118) -> (24.2324, -100.9118)
  line L74 (-24.2324, 17.4823) -> (-24.2324, -17.4824)
  line L75 (-24.2324, -17.4824) -> (-100.9117, -17.4824)
  line L76 (-100.9117, -17.4824) -> (-100.9117, 17.4823)
  line L77 (-100.9117, 17.4823) -> (-24.2324, 17.4823)
  line L78 (-59.1972, 59.197) -> (-59.1973, 100.9118)
  line L79 (-59.1973, 100.9118) -> (-24.2324, 100.9119)
  line L80 (-24.2324, 100.9119) -> (-24.2324, 24.2323)
  line L81 (-24.2324, 24.2323) -> (-107.6617, 24.2323)
  line L82 (-107.6617, 24.2323) -> (-107.6616, -17.4824)
  line L83 (-107.6616, -17.4824) -> (-124.8909, -17.4824)
  arc A8 (-104.0798, 59.197) -> (-124.8909, -17.4824) centre (-37.6354, -0.0001) ccw
  line L84 (-104.0798, 59.197) -> (-59.1972, 59.197)
  line L85 (-79.2873, -65.9474) -> (-83.2873, -65.9474)
  line L86 (-83.2873, -65.9474) -> (-83.2873, -59.1973)
  line L87 (-83.2873, -59.1973) -> (-79.2873, -59.1973)
  line L88 (-79.2873, -59.1973) -> (-79.2873, -65.9474)
  dimension "d74" = 4
  measures "d74" distance of L85.start L85.end
extrude "Extrude9" add sketch "Sketch9" along normal blind 7 contours L12 L53 L85 L86 L87 L88 bodies 1
extrude "Extrude10" cut 1 faces at (22.0093, 32.4, -63.6974) along direction (0, -1, 0) blind 7 on bodies 2 bodies 2